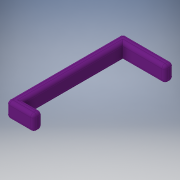
# Autodesk Inventor part: Bumpers_2020
Saved by Autodesk Inventor 2017 (Build 210142000, 142)
## iProperties
Created: 2020-01-31
Part Number: Bumpers_2020
Material: Generic
Document SubType Name: Sheet Metal
Designer: S346905847
Density: 1 g/cm^3
Sheet Metal Rule: Default
Appearance: Default
Author: S346905847
Autodesk Inventor part; units mm, degrees
ref_plane "YZ Plane" through (0, 0, 0) normal (1, 0, 0) x (0, 1, 0)
ref_plane "XZ Plane" through (0, 0, 0) normal (0, 1, 0) x (-1, 0, 0)
ref_plane "XY Plane" through (0, 0, 0) normal (0, 0, 1) x (1, 0, 0)
sketch "Sketch1" plane through (0, 0, 0) normal (0, 1, 0) x (-1, 0, 0)
  line L0 (0, 0) -> (-69.85, 0)
  line L1 (-69.85, 0) -> (-69.85, -946.15)
  line L2 (-69.85, -946.15) -> (0, -946.15)
  line L3 (0, -946.15) -> (0, 0)
  dimension "d0" = 946.15
  dimension "d1" = 69.85
  constraints: 8 end point, 2 parallel, 1 horizontal, 1 perpendicular
  measures "d0" distance of L2.end L0.start
  measures "d1" distance of L1.end L2.end
extrude "Extrusion1" add sketch "Sketch1" along normal blind 127
sketch "Sketch2" plane through (69.85, 0, 0) normal (1, 0, 0) x (0, 0, -1)
  line L0 (0, 127) -> (69.85, 127)
  line L1 (69.85, 127) -> (69.85, 0)
  line L2 (69.85, 0) -> (0, 0)
  line L3 (0, 0) -> (0, 127)
  point P0 (946.15, 127)
  dimension "d4" = 69.85
  constraints: 8 end point, 2 parallel, 1 horizontal, 1 perpendicular
  measures "d4" distance of L0.end L0.start
extrude "Extrusion2" add sketch "Sketch2" along normal blind 152.4
sketch "Sketch3" plane through (69.85, 0, -946.15) normal (1, 0, 0) x (0, 0, -1)
  line L0 (0, 0) -> (0, 127) projected
  line L1 (-876.3, 127) -> (0, 127) projected
  line L2 (0, 0) -> (-69.85, 0)
  line L3 (-69.85, 0) -> (-69.85, 127)
  line L4 (-69.85, 127) -> (0, 127)
  line L5 (0, 127) -> (0, 0)
  point P0 (-946.15, 0)
  dimension "d8" = 69.85
  constraints: 8 end point, 2 parallel, 1 horizontal, 1 perpendicular, 1 point on line
  measures "d8" distance of L3.end L4.end
extrude "Extrusion3" add sketch "Sketch3" along normal blind 342.9
fillet "Fillet1" radius 25.4 1 edges at (222.25, 127, -34.925)
fillet "Fillet2" radius 25.4 1 edges at (412.75, 127, -911.225)
fillet "Fillet6" radius 25.4 3 edges at (193.675, 127, -946.15) (405.3105, 119.5605, -946.15) (412.75, 50.8, -946.15)
fillet "Fillet7" radius 25.4 3 edges at (0, 127, -460.375) (0, 119.5605, -938.7105) (0, 50.8, -946.15)
fillet "Fillet8" radius 25.4 5 edges at (214.8105, 119.5605, 0) (222.25, 50.8, 0) (7.4395, 119.5605, 0) (0, 50.8, 0) (111.125, 127, 0)
sketch "Sketch4" plane through (412.75, 0, -946.15) normal (1, 0, 0) x (0, 0, -1)
  line L0 (-25.4, 101.6) -> (-25.4, 0) projected
  line L1 (-69.85, 101.6) -> (-25.4, 101.6) projected
  line L2 (-25.4, 0) -> (-69.85, 0)
  line L3 (-69.85, 0) -> (-69.85, 101.6)
  line L4 (-69.85, 101.6) -> (-25.4, 101.6)
  line L5 (-25.4, 101.6) -> (-25.4, 0)
  point P0 (-946.15, 0)
  constraints: 8 end point, 2 parallel, 1 horizontal, 1 perpendicular
extrude "Extrusion4" add sketch "Sketch4" along normal blind 12.7
sketch "Sketch5" plane through (425.45, 0, -946.15) normal (1, 0, 0) x (0, 0, -1)
  line L0 (-69.85, 101.6) -> (-69.85, 0) projected
  line L1 (-69.85, 101.6) -> (-25.4, 101.6)
  line L2 (-25.4, 101.6) -> (-25.4, 0)
  line L3 (-25.4, 0) -> (-69.85, 0)
  line L4 (-69.85, 0) -> (-69.85, 101.6)
  point P0 (-946.15, 0)
  constraints: 8 end point, 2 parallel, 1 horizontal, 1 perpendicular
extrude "Extrusion5" cut sketch "Sketch5" against normal blind 12.7
fillet "Fillet9" radius 25.4 19 edges at (214.8105, 0, -7.4395) (222.25, 0, -47.625) (7.4395, 0, -7.4395) (0, 0, -473.075) (7.4395, 0, -938.7105) (206.375, 0, -946.15) (405.3105, 0, -938.7105) (412.75, 0, -898.525) (111.125, 0, 0) (146.05, 0, -69.85) (69.85, 0, -473.075) (241.3, 0, -876.3) (405.3105, 119.5605, -876.3) (228.6, 127, -876.3) (412.75, 50.8, -876.3) (214.8105, 119.5605, -69.85) (133.35, 127, -69.85) (222.25, 50.8, -69.85) (69.85, 127, -473.075)
equation "\"BendRadius\" = Thickness"
equation "\"BendReliefWidth\" = Thickness"
equation "\"BendReliefDepth\" = 0.5 * Thickness"
equation "\"CornerReliefSize\" = 4 * Thickness"
equation "\"MinimumRemnant\" = 2 * Thickness"
equation "\"TransitionRadius\" = BendRadius"
equation "\"JacobiRadiusSize\" = BendRadius"
equation "\"GapSize\" = Thickness"
equation "\"Thickness\" = 3.048"
body "Solid1"
